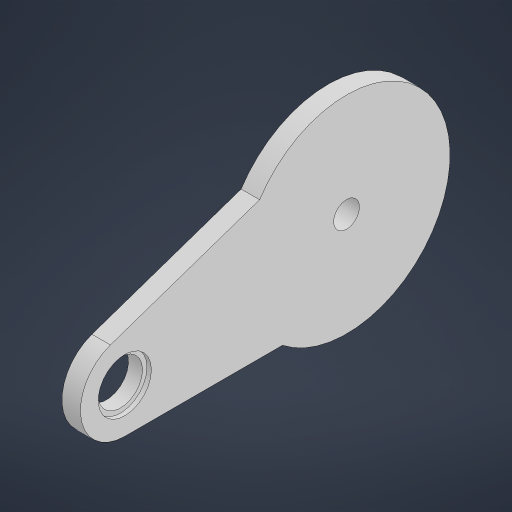
# Autodesk Inventor part: Main_Frame
Saved by Autodesk Inventor 2024.2 (Build 282272000, 272)
## iProperties
Created: 2024-03-05
Part Number: Main_Frame
Material: 一般
Document SubType Name: Modeling
Designer: Hanaoka
Density: 1 g/cm^3
Appearance: 既定
Author: Hanaoka
Autodesk Inventor part; units mm, degrees
ref_plane "YZ Plane" through (0, 0, 0) normal (1, 0, 0) x (0, 1, 0)
ref_plane "XZ Plane" through (0, 0, 0) normal (0, 1, 0) x (-1, 0, 0)
ref_plane "XY Plane" through (0, 0, 0) normal (0, 0, 1) x (1, 0, 0)
sketch "スケッチ1" plane through (0, 0, 0) normal (1, 0, 0) x (0, 1, 0)
  circle A0 centre (0, 0) radius 6
  circle A1 centre (5, -30) radius 11
  line L0 (-6, 0) -> (-6, -30)
  line L1 (5.6757, 1.9459) -> (15.4054, -26.4324)
  circle A2 centre (5, -30) radius 14
  circle A3 centre (0, 0) radius 3
  circle A4 centre (5, -30) radius 1.75
  point P0 (-6, -21.3397)
  point P1 (12.5967, -18.2403)
  dimension "d0" = 12
  dimension "d1" = 22
  dimension "d2" = 30
  dimension "d3" = 28
  dimension "d4" = 6
  dimension "d5" = 3.5
  constraints: 5 centre point, 4 coincident, 4 end point, 4 point on circle, 4 tangent, 1 vertical
  measures "d0" diameter of A0
  measures "d1" diameter of A1
  measures "d2" distance of L0.start L0.end
  measures "d3" diameter of A2
  measures "d4" diameter of A3
  measures "d5" diameter of A4
extrude "押し出し1" add sketch "スケッチ1" along normal blind 2.5
sketch "スケッチ2" plane through (2.5, 0, 0) normal (1, 0, 0) x (0, 0, -1)
  circle A0 centre (0, 0) radius 3.6
  circle A1 centre (0, 0) radius 3 projected
  dimension "d8" = 7.2
  constraints: 1 centre point, 1 coincident
  measures "d8" diameter of A0
extrude "押し出し2" cut sketch "スケッチ2" against normal blind 0.6
